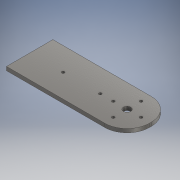
# Autodesk Inventor part: laterales
Saved by Autodesk Inventor 2018 (Build 220112000, 112)
## iProperties
Created: 2019-04-02
Part Number: laterales
Material: Acero, galvanizado
Document SubType Name: Modeling
Designer: Victor Hernandez
Density: 7.85 g/cm^3
Appearance: Galvanizado
Author: Victor Hernandez
Autodesk Inventor part; units mm, degrees
ref_plane "YZ Plane" through (0, 0, 0) normal (1, 0, 0) x (0, 1, 0)
ref_plane "XZ Plane" through (0, 0, 0) normal (0, 1, 0) x (-1, 0, 0)
ref_plane "XY Plane" through (0, 0, 0) normal (0, 0, 1) x (1, 0, 0)
sketch "Boceto1" plane through (0, 0, 0) normal (0, 0, 1) x (1, 0, 0)
  line L0 (-32.5, -12.5) -> (32.5, -12.5)
  line L1 (32.5, -12.5) -> (32.5, 12.5)
  line L2 (32.5, 12.5) -> (-32.5, 12.5)
  line L3 (-32.5, 12.5) -> (-32.5, -12.5)
  line L4 (-32.5, -12.5) -> (32.5, 12.5) construction
  line L5 (32.5, -12.5) -> (-32.5, 12.5) construction
  circle A0 centre (-14.5, 0) radius 0.75
  circle A1 centre (5.5, 0) radius 0.75
  circle A2 centre (27.5, 0) radius 0.75
  circle A3 centre (20, 0) radius 2
  circle A4 centre (12.5, 0) radius 0.75
  circle A5 centre (20, 7.5) radius 0.75
  circle A6 centre (20, -7.5) radius 0.75
  point P0 (0, 0)
  dimension "d0" = 65
  dimension "d1" = 25
  dimension "d11" = 1.5
  dimension "d12" = 1.5
  dimension "d13" = 1.5
  dimension "d14" = 4
  dimension "d15" = 1.5
  dimension "d16" = 1.5
  dimension "d17" = 1.5
  constraints: 12 end point, 7 centre point, 2 midpoint, 2 parallel, 1 horizontal, 1 perpendicular
  measures "d0" distance of L2.end L1.end
  measures "d1" distance of L1.end L0.end
  measures "d11" diameter of A0
  measures "d12" diameter of A1
  measures "d13" diameter of A2
  measures "d14" diameter of A3
  measures "d15" diameter of A4
  measures "d16" diameter of A5
  measures "d17" diameter of A6
extrude "Extrusión1" add sketch "Boceto1" along normal blind 2
fillet "Empalme1" radius 12 1 edges at (32.5, 12.5, 1)
fillet "Empalme2" radius 12 1 edges at (32.5, -12.5, 1)
